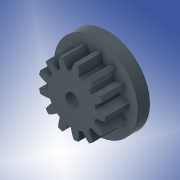
# Autodesk Inventor part: BA006
Saved by Autodesk Inventor 2017 (Build 210142000, 142)
## iProperties
Created: 2017-06-15
Part Number: BA006
Material: ABS Plastic
Document SubType Name: Modeling
Designer: zallen
Density: 1.06 g/cm^3
Appearance: CR Dark Blue
Author: zallen
Autodesk Inventor part; units mm, degrees
ref_plane "YZ Plane" through (0, 0, 0) normal (1, 0, 0) x (0, 1, 0)
ref_plane "XZ Plane" through (0, 0, 0) normal (0, 1, 0) x (-1, 0, 0)
ref_plane "XY Plane" through (0, 0, 0) normal (0, 0, 1) x (1, 0, 0)
sketch "Sketch1" plane through (0, 0, 0) normal (0, 0, 1) x (1, 0, 0)
  circle A0 centre (0, 0) radius 10
  arc A1 (13.8638, 0.9) -> (9.8638, 1.6449) centre (9.1431, -13.3378) ccw
  arc A2 (9.8638, -1.6449) -> (13.8638, -0.9) centre (9.1431, 13.3378) ccw
  arc A3 (13.8638, -0.9) -> (13.8638, 0.9) centre (-6.1159, 0) ccw
  line L0 (0, 0) -> (21.7354, 0) construction
  arc A4 (9.8638, -1.6449) -> (9.8638, 1.6449) centre (0, 0) ccw
  arc A5 (11.8575, 7.2397) -> (7.9696, 6.0404) centre (14.2942, -7.561) ccw
  arc A6 (12.694, 5.6459) -> (11.8575, 7.2397) centre (-5.4154, -2.8422) ccw
  arc A7 (9.4984, 3.1275) -> (12.694, 5.6459) centre (1.8975, 16.0591) ccw
  circle A8 centre (0, 0) radius 10
  arc A9 (9.4984, 3.1275) -> (7.9696, 6.0404) centre (0, 0) ccw
  arc A10 (7.1348, 11.9209) -> (4.2496, 9.0521) centre (16.1707, -0.0521) ccw
  arc A11 (8.6162, 10.8984) -> (7.1348, 11.9209) centre (-3.4743, -5.0333) ccw
  arc A12 (6.957, 7.1834) -> (8.6162, 10.8984) centre (-5.7829, 15.1014) ccw
  circle A13 centre (0, 0) radius 10
  arc A14 (6.957, 7.1834) -> (4.2496, 9.0521) centre (0, 0) ccw
  arc A15 (0.7777, 13.8712) -> (-0.4439, 9.9901) centre (14.3427, 7.4688) ccw
  arc A16 (2.5645, 13.6542) -> (0.7777, 13.8712) centre (-0.7372, -6.0714) ccw
  arc A17 (2.8218, 9.5936) -> (2.5645, 13.6542) centre (-12.1385, 10.6842) ccw
  circle A18 centre (0, 0) radius 10
  arc A19 (2.8218, 9.5936) -> (-0.4439, 9.9901) centre (0, 0) ccw
  arc A20 (-5.7577, 12.6437) -> (-5.0357, 8.6395) centre (9.2289, 13.2786) ccw
  arc A21 (-4.0747, 13.282) -> (-5.7577, 12.6437) centre (2.1687, -5.7185) ccw
  arc A22 (-1.9598, 9.8061) -> (-4.0747, 13.282) centre (-15.7133, 3.8193) ccw
  circle A23 centre (0, 0) radius 10
  arc A24 (-1.9598, 9.8061) -> (-5.0357, 8.6395) centre (0, 0) ccw
  arc A25 (-10.974, 8.5197) -> (-8.4739, 5.3097) centre (2.0009, 16.0465) ccw
  arc A26 (-9.7804, 9.8671) -> (-10.974, 8.5197) centre (4.5779, -4.0556) ccw
  arc A27 (-6.2924, 7.7721) -> (-9.7804, 9.8671) centre (-15.6884, -3.9205) ccw
  circle A28 centre (0, 0) radius 10
  arc A29 (-6.2924, 7.7721) -> (-8.4739, 5.3097) centre (0, 0) ccw
  arc A30 (-13.6763, 2.444) -> (-9.9708, 0.7635) centre (-5.6855, 15.1383) ccw
  arc A31 (-13.2456, 4.1917) -> (-13.6763, 2.444) centre (5.9382, -1.4636) ccw
  arc A32 (-9.1835, 3.9576) -> (-13.2456, 4.1917) centre (-12.0694, -10.7621) ccw
  circle A33 centre (0, 0) radius 10
  arc A34 (-9.1835, 3.9576) -> (-9.9708, 0.7635) centre (0, 0) ccw
  arc A35 (-13.2456, -4.1917) -> (-9.1835, -3.9576) centre (-12.0694, 10.7621) ccw
  arc A36 (-13.6763, -2.444) -> (-13.2456, -4.1917) centre (5.9382, 1.4636) ccw
  arc A37 (-9.9708, -0.7635) -> (-13.6763, -2.444) centre (-5.6855, -15.1383) ccw
  circle A38 centre (0, 0) radius 10
  arc A39 (-9.9708, -0.7635) -> (-9.1835, -3.9576) centre (0, 0) ccw
  arc A40 (-9.7804, -9.8671) -> (-6.2924, -7.7721) centre (-15.6884, 3.9205) ccw
  arc A41 (-10.974, -8.5197) -> (-9.7804, -9.8671) centre (4.5779, 4.0556) ccw
  arc A42 (-8.4739, -5.3097) -> (-10.974, -8.5197) centre (2.0009, -16.0465) ccw
  circle A43 centre (0, 0) radius 10
  arc A44 (-8.4739, -5.3097) -> (-6.2924, -7.7721) centre (0, 0) ccw
  arc A45 (-4.0747, -13.282) -> (-1.9598, -9.8061) centre (-15.7133, -3.8193) ccw
  arc A46 (-5.7577, -12.6437) -> (-4.0747, -13.282) centre (2.1687, 5.7185) ccw
  arc A47 (-5.0357, -8.6395) -> (-5.7577, -12.6437) centre (9.2289, -13.2786) ccw
  circle A48 centre (0, 0) radius 10
  arc A49 (-5.0357, -8.6395) -> (-1.9598, -9.8061) centre (0, 0) ccw
  arc A50 (2.5645, -13.6542) -> (2.8218, -9.5936) centre (-12.1385, -10.6842) ccw
  arc A51 (0.7777, -13.8712) -> (2.5645, -13.6542) centre (-0.7372, 6.0714) ccw
  arc A52 (-0.4439, -9.9901) -> (0.7777, -13.8712) centre (14.3427, -7.4688) ccw
  circle A53 centre (0, 0) radius 10
  arc A54 (-0.4439, -9.9901) -> (2.8218, -9.5936) centre (0, 0) ccw
  arc A55 (8.6162, -10.8984) -> (6.957, -7.1834) centre (-5.7829, -15.1014) ccw
  arc A56 (7.1348, -11.9209) -> (8.6162, -10.8984) centre (-3.4743, 5.0333) ccw
  arc A57 (4.2496, -9.0521) -> (7.1348, -11.9209) centre (16.1707, 0.0521) ccw
  circle A58 centre (0, 0) radius 10
  arc A59 (4.2496, -9.0521) -> (6.957, -7.1834) centre (0, 0) ccw
  arc A60 (12.694, -5.6459) -> (9.4984, -3.1275) centre (1.8975, -16.0591) ccw
  arc A61 (11.8575, -7.2397) -> (12.694, -5.6459) centre (-5.4154, 2.8422) ccw
  arc A62 (7.9696, -6.0404) -> (11.8575, -7.2397) centre (14.2942, 7.561) ccw
  circle A63 centre (0, 0) radius 10
  arc A64 (7.9696, -6.0404) -> (9.4984, -3.1275) centre (0, 0) ccw
  dimension "d0" = 20
  dimension "d3" = 15
  dimension "d4" = 15
  dimension "d5" = 4
  dimension "d6" = 20
  dimension "d7" = 1.8
  dimension "d10" = 360
  constraints: 130 point on circle, 65 centre point, 2 end point, 2 symmetric about line, 2 vertical alignment, 1 coincident, 1 concentric, 1 horizontal, 183 other
  measures "d0" diameter of A0
  measures "d3" radius of A1
  measures "d4" radius of A2
  measures "d5" horizontal distance of A1.start A0.start
  measures "d6" radius of A3
  measures "d7" distance of A2.end A1.start
extrude "Extrusion1" add sketch "Sketch1" along normal blind 10
sketch "Sketch2" plane through (0, 0, 10) normal (0, 0, 1) x (1, 0, 0)
  circle A0 centre (0, 0) radius 2.75
  dimension "d14" = 5.5
  constraints: 1 centre point, 1 coincident
  measures "d14" diameter of A0
extrude "Extrusion2" cut sketch "Sketch2" against normal through all
sketch "Sketch3" plane through (0, 0, 0) normal (0, 0, -1) x (-1, 0, 0)
  circle A0 centre (0, 0) radius 17.5
  circle A1 centre (0, 0) radius 3.2083
  dimension "d17" = 35
  constraints: 2 centre point, 2 coincident
  measures "d17" diameter of A0
extrude "Extrusion3" add sketch "Sketch3" along normal blind 5
body "Solid1"
